Autodesk Inventor part; units mm, degrees
(part 2 of 2)
  line L983 (36.3398, 14.9098) -> (36.7208, 14.9098)
  line L984 (36.5303, 14.7193) -> (36.5303, 15.1003)
  line L985 (36.3398, 15.9918) -> (36.7208, 15.9918)
  line L986 (36.5303, 15.8013) -> (36.5303, 16.1823)
  line L987 (35.2146, 14.9098) -> (35.5956, 14.9098)
  line L988 (35.4051, 14.7193) -> (35.4051, 15.1003)
  line L989 (35.2146, 15.9918) -> (35.5956, 15.9918)
  line L990 (35.4051, 15.8013) -> (35.4051, 16.1823)
  line L991 (34.0893, 17.0713) -> (34.4703, 17.0713)
  line L992 (34.2798, 16.8808) -> (34.2798, 17.2618)
  line L993 (36.3398, 17.0713) -> (36.7208, 17.0713)
  line L994 (36.5303, 16.8808) -> (36.5303, 17.2618)
  line L995 (34.0893, 15.9918) -> (34.4703, 15.9918)
  line L996 (34.2798, 15.8013) -> (34.2798, 16.1823)
  line L997 (35.2146, 17.0713) -> (35.5956, 17.0713)
  line L998 (35.4051, 16.8808) -> (35.4051, 17.2618)
  line L999 (37.465, 17.0713) -> (37.846, 17.0713)
  line L1000 (37.6555, 16.8808) -> (37.6555, 17.2618)
  line L1001 (38.5902, 17.0713) -> (38.9712, 17.0713)
  line L1002 (38.7807, 16.8808) -> (38.7807, 17.2618)
  line L1003 (34.0893, 14.9098) -> (34.4703, 14.9098)
  line L1004 (34.2798, 14.7193) -> (34.2798, 15.1003)
  line L1005 (34.0893, 13.7617) -> (34.4703, 13.7617)
  line L1006 (34.2798, 13.5712) -> (34.2798, 13.9522)
  line L1007 (38.5902, 11.6002) -> (38.9712, 11.6002)
  line L1008 (38.7807, 11.4097) -> (38.7807, 11.7907)
  line L1009 (37.465, 11.6002) -> (37.846, 11.6002)
  line L1010 (37.6555, 11.4097) -> (37.6555, 11.7907)
  line L1011 (35.2146, 11.6002) -> (35.5956, 11.6002)
  line L1012 (35.4051, 11.4097) -> (35.4051, 11.7907)
  line L1013 (34.0893, 12.6822) -> (34.4703, 12.6822)
  line L1014 (34.2798, 12.4917) -> (34.2798, 12.8727)
  line L1015 (36.3398, 11.6002) -> (36.7208, 11.6002)
  line L1016 (36.5303, 11.4097) -> (36.5303, 11.7907)
  line L1017 (34.0893, 11.6002) -> (34.4703, 11.6002)
  line L1018 (34.2798, 11.4097) -> (34.2798, 11.7907)
  line L1019 (35.2146, 12.6822) -> (35.5956, 12.6822)
  line L1020 (35.4051, 12.4917) -> (35.4051, 12.8727)
  line L1021 (35.2146, 13.7617) -> (35.5956, 13.7617)
  line L1022 (35.4051, 13.5712) -> (35.4051, 13.9522)
  line L1023 (36.3398, 12.6822) -> (36.7208, 12.6822)
  line L1024 (36.5303, 12.4917) -> (36.5303, 12.8727)
  line L1025 (36.3398, 13.7617) -> (36.7208, 13.7617)
  line L1026 (36.5303, 13.5712) -> (36.5303, 13.9522)
  line L1027 (37.465, 12.6822) -> (37.846, 12.6822)
  line L1028 (37.6555, 12.4917) -> (37.6555, 12.8727)
  line L1029 (37.465, 13.7617) -> (37.846, 13.7617)
  line L1030 (37.6555, 13.5712) -> (37.6555, 13.9522)
  line L1031 (38.5902, 12.6822) -> (38.9712, 12.6822)
  line L1032 (38.7807, 12.4917) -> (38.7807, 12.8727)
  line L1033 (38.5902, 13.7617) -> (38.9712, 13.7617)
  line L1034 (38.7807, 13.5712) -> (38.7807, 13.9522)
  line L1035 (38.5902, 10.5207) -> (38.9712, 10.5207)
  line L1036 (38.7807, 10.3302) -> (38.7807, 10.7112)
  line L1037 (37.465, 10.5207) -> (37.846, 10.5207)
  line L1038 (37.6555, 10.3302) -> (37.6555, 10.7112)
  line L1039 (36.3398, 10.5207) -> (36.7208, 10.5207)
  line L1040 (36.5303, 10.3302) -> (36.5303, 10.7112)
  line L1041 (35.2146, 10.5207) -> (35.5956, 10.5207)
  line L1042 (35.4051, 10.3302) -> (35.4051, 10.7112)
  line L1043 (34.0893, 9.4412) -> (34.4703, 9.4412)
  line L1044 (34.2798, 9.2507) -> (34.2798, 9.6317)
  line L1045 (36.3398, 9.4412) -> (36.7208, 9.4412)
  line L1046 (36.5303, 9.2507) -> (36.5303, 9.6317)
  line L1047 (34.0893, 10.5207) -> (34.4703, 10.5207)
  line L1048 (34.2798, 10.3302) -> (34.2798, 10.7112)
  line L1049 (35.2146, 9.4412) -> (35.5956, 9.4412)
  line L1050 (35.4051, 9.2507) -> (35.4051, 9.6317)
  line L1051 (37.465, 9.4412) -> (37.846, 9.4412)
  line L1052 (37.6555, 9.2507) -> (37.6555, 9.6317)
  line L1053 (38.5902, 9.4412) -> (38.9712, 9.4412)
  line L1054 (38.7807, 9.2507) -> (38.7807, 9.6317)
  line L1055 (38.5902, 19.2303) -> (38.9712, 19.2303)
  line L1056 (38.7807, 19.0398) -> (38.7807, 19.4208)
  line L1057 (37.465, 19.2303) -> (37.846, 19.2303)
  line L1058 (37.6555, 19.0398) -> (37.6555, 19.4208)
  line L1059 (35.2146, 19.2303) -> (35.5956, 19.2303)
  line L1060 (35.4051, 19.0398) -> (35.4051, 19.4208)
  line L1061 (34.0893, 18.1508) -> (34.4703, 18.1508)
  line L1062 (34.2798, 17.9603) -> (34.2798, 18.3413)
  line L1063 (36.3398, 19.2303) -> (36.7208, 19.2303)
  line L1064 (36.5303, 19.0398) -> (36.5303, 19.4208)
  line L1065 (34.0893, 19.2303) -> (34.4703, 19.2303)
  line L1066 (34.2798, 19.0398) -> (34.2798, 19.4208)
  line L1067 (35.2146, 18.1508) -> (35.5956, 18.1508)
  line L1068 (35.4051, 17.9603) -> (35.4051, 18.3413)
  line L1069 (36.3398, 18.1508) -> (36.7208, 18.1508)
  line L1070 (36.5303, 17.9603) -> (36.5303, 18.3413)
  line L1071 (37.465, 18.1508) -> (37.846, 18.1508)
  line L1072 (37.6555, 17.9603) -> (37.6555, 18.3413)
  line L1073 (38.5902, 18.1508) -> (38.9712, 18.1508)
  line L1074 (38.7807, 17.9603) -> (38.7807, 18.3413)
  line L1075 (24.1935, 38.735) -> (24.5745, 38.735)
  line L1076 (24.384, 38.5445) -> (24.384, 38.9255)
  line L1077 (21.3995, 35.56) -> (21.7805, 35.56)
  line L1078 (21.59, 35.3695) -> (21.59, 35.7505)
  line L1079 (3.8735, 27.94) -> (4.2545, 27.94)
  line L1080 (4.064, 27.7495) -> (4.064, 28.1305)
  line L1081 (3.8735, 17.653) -> (4.2545, 17.653)
  line L1082 (4.064, 17.4625) -> (4.064, 17.8435)
  line L1083 (3.1115, 20.574) -> (3.4925, 20.574)
  line L1084 (3.302, 20.3835) -> (3.302, 20.7645)
  line L1085 (4.8895, 27.94) -> (5.2705, 27.94)
  line L1086 (5.08, 27.7495) -> (5.08, 28.1305)
  line L1087 (4.6355, 18.415) -> (5.0165, 18.415)
  line L1088 (4.826, 18.2245) -> (4.826, 18.6055)
  line L1089 (3.8735, 10.541) -> (4.2545, 10.541)
  line L1090 (4.064, 10.3505) -> (4.064, 10.7315)
  line L1091 (10.6045, 34.29) -> (10.9855, 34.29)
  line L1092 (10.795, 34.0995) -> (10.795, 34.4805)
  line L1093 (9.4615, 8.128) -> (9.8425, 8.128)
  line L1094 (9.652, 7.9375) -> (9.652, 8.3185)
  line L1095 (7.8105, 13.081) -> (8.1915, 13.081)
  line L1096 (8.001, 12.8905) -> (8.001, 13.2715)
  line L1097 (47.8155, 27.94) -> (48.1965, 27.94)
  line L1098 (48.006, 27.7495) -> (48.006, 28.1305)
  line L1099 (12.446, 26.4414) -> (12.954, 26.4414)
  line L1100 (12.7, 26.1874) -> (12.7, 26.6954)
  line L1101 (19.2405, 47.5107) -> (19.6215, 47.5107)
  line L1102 (19.431, 47.3202) -> (19.431, 47.7012)
  line L1103 (18.7325, 11.303) -> (19.1135, 11.303)
  line L1104 (18.923, 11.1125) -> (18.923, 11.4935)
  line L1105 (18.2245, 10.414) -> (18.6055, 10.414)
  line L1106 (18.415, 10.2235) -> (18.415, 10.6045)
  line L1107 (18.2245, 9.398) -> (18.6055, 9.398)
  line L1108 (18.415, 9.2075) -> (18.415, 9.5885)
  line L1109 (23.5585, 11.176) -> (23.9395, 11.176)
  line L1110 (23.749, 10.9855) -> (23.749, 11.3665)
  line L1111 (18.0975, 6.223) -> (18.4785, 6.223)
  line L1112 (18.288, 6.0325) -> (18.288, 6.4135)
  line L1113 (16.7005, 50.038) -> (17.0815, 50.038)
  line L1114 (16.891, 49.8475) -> (16.891, 50.2285)
  line L1115 (9.7155, 43.053) -> (10.0965, 43.053)
  line L1116 (9.906, 42.8625) -> (9.906, 43.2435)
  line L1117 (12.5095, 43.053) -> (12.8905, 43.053)
  line L1118 (12.7, 42.8625) -> (12.7, 43.2435)
  line L1119 (5.3975, 26.035) -> (5.7785, 26.035)
  line L1120 (5.588, 25.8445) -> (5.588, 26.2255)
  line L1121 (6.1595, 25.4) -> (6.5405, 25.4)
  line L1122 (6.35, 25.2095) -> (6.35, 25.5905)
  line L1123 (7.8105, 25.4) -> (8.1915, 25.4)
  line L1124 (8.001, 25.2095) -> (8.001, 25.5905)
  line L1125 (7.0485, 24.638) -> (7.4295, 24.638)
  line L1126 (7.239, 24.4475) -> (7.239, 24.8285)
  line L1127 (8.5725, 26.035) -> (8.9535, 26.035)
  line L1128 (8.763, 25.8445) -> (8.763, 26.2255)
  line L1129 (28.7655, 14.3358) -> (29.1465, 14.3358)
  line L1130 (28.956, 14.1453) -> (28.956, 14.5263)
  line L1131 (28.4226, -3.4544) -> (27.4091, -3.4544)
  line L1132 (27.4091, -3.4544) -> (28.4226, -2.4384)
  line L1133 (28.4226, -2.4384) -> (28.4226, -2.1844)
  line L1134 (28.4226, -2.1844) -> (28.1711, -1.9304)
  line L1135 (28.1711, -1.9304) -> (27.6631, -1.9304)
  line L1136 (27.6631, -1.9304) -> (27.4091, -2.1844)
  line L1137 (29.9466, -1.9304) -> (28.9306, -1.9304)
  line L1138 (28.9306, -1.9304) -> (28.9306, -2.6924)
  line L1139 (28.9306, -2.6924) -> (29.4386, -2.4384)
  line L1140 (29.4386, -2.4384) -> (29.6926, -2.4384)
  line L1141 (29.6926, -2.4384) -> (29.9466, -2.6924)
  line L1142 (29.9466, -2.6924) -> (29.9466, -3.2004)
  line L1143 (29.9466, -3.2004) -> (29.6926, -3.4544)
  line L1144 (29.6926, -3.4544) -> (29.1846, -3.4544)
  line L1145 (29.1846, -3.4544) -> (28.9306, -3.2004)
  line L1146 (31.4706, -1.9304) -> (30.9626, -2.1844)
  line L1147 (30.9626, -2.1844) -> (30.4546, -2.6924)
  line L1148 (30.4546, -2.6924) -> (30.4546, -3.2004)
  line L1149 (30.4546, -3.2004) -> (30.7086, -3.4544)
  line L1150 (30.7086, -3.4544) -> (31.2166, -3.4544)
  line L1151 (31.2166, -3.4544) -> (31.4706, -3.2004)
  line L1152 (31.4706, -3.2004) -> (31.4706, -2.9464)
  line L1153 (31.4706, -2.9464) -> (31.2166, -2.6924)
  line L1154 (31.2166, -2.6924) -> (30.4546, -2.6924)
  line L1155 (31.9786, -2.1844) -> (32.2326, -1.9304)
  line L1156 (32.2326, -1.9304) -> (32.7406, -1.9304)
  line L1157 (32.7406, -1.9304) -> (32.9946, -2.1844)
  line L1158 (32.9946, -2.1844) -> (32.9946, -3.2004)
  line L1159 (32.9946, -3.2004) -> (32.7406, -3.4544)
  line L1160 (32.7406, -3.4544) -> (32.2326, -3.4544)
  line L1161 (32.2326, -3.4544) -> (31.9786, -3.2004)
  line L1162 (31.9786, -3.2004) -> (31.9786, -2.1844)
  line L1163 (33.5026, -3.4544) -> (33.5026, -2.4384)
  line L1164 (33.5026, -2.4384) -> (33.7566, -2.4384)
  line L1165 (33.7566, -2.4384) -> (34.0106, -2.6924)
  line L1166 (34.0106, -2.6924) -> (34.0106, -3.4544)
  line L1167 (34.0106, -3.4544) -> (34.0106, -2.6924)
  line L1168 (34.0106, -2.6924) -> (34.2646, -2.4384)
  line L1169 (34.2646, -2.4384) -> (34.5186, -2.6924)
  line L1170 (34.5186, -2.6924) -> (34.5186, -3.4544)
  line L1171 (35.0266, -3.4544) -> (35.5346, -3.4544)
  line L1172 (35.5346, -3.4544) -> (35.2806, -3.4544)
  line L1173 (35.2806, -3.4544) -> (35.2806, -2.4384)
  line L1174 (35.2806, -2.4384) -> (35.0266, -2.4384)
  line L1175 (36.2941, -3.4544) -> (36.8021, -3.4544)
  line L1176 (36.8021, -3.4544) -> (36.5481, -3.4544)
  line L1177 (36.5481, -3.4544) -> (36.5481, -1.9304)
  line L1178 (36.5481, -1.9304) -> (36.2941, -1.9304)
  line L1179 (-1.6256, 21.5646) -> (-1.6256, 20.5511)
  line L1180 (-1.6256, 20.5511) -> (-2.6416, 21.5646)
  line L1181 (-2.6416, 21.5646) -> (-2.8956, 21.5646)
  line L1182 (-2.8956, 21.5646) -> (-3.1496, 21.3106)
  line L1183 (-3.1496, 21.3106) -> (-3.1496, 20.8051)
  line L1184 (-3.1496, 20.8051) -> (-2.8956, 20.5511)
  line L1185 (-2.8956, 22.0726) -> (-3.1496, 22.3266)
  line L1186 (-3.1496, 22.3266) -> (-3.1496, 22.8346)
  line L1187 (-3.1496, 22.8346) -> (-2.8956, 23.0886)
  line L1188 (-2.8956, 23.0886) -> (-1.8796, 23.0886)
  line L1189 (-1.8796, 23.0886) -> (-1.6256, 22.8346)
  line L1190 (-1.6256, 22.8346) -> (-1.6256, 22.3266)
  line L1191 (-1.6256, 22.3266) -> (-1.8796, 22.0726)
  line L1192 (-1.8796, 22.0726) -> (-2.8956, 22.0726)
  line L1193 (-1.6256, 24.6126) -> (-1.6256, 23.5966)
  line L1194 (-1.6256, 23.5966) -> (-2.6416, 24.6126)
  line L1195 (-2.6416, 24.6126) -> (-2.8956, 24.6126)
  line L1196 (-2.8956, 24.6126) -> (-3.1496, 24.3586)
  line L1197 (-3.1496, 24.3586) -> (-3.1496, 23.8506)
  line L1198 (-3.1496, 23.8506) -> (-2.8956, 23.5966)
  line L1199 (-2.8956, 25.1206) -> (-3.1496, 25.3746)
  line L1200 (-3.1496, 25.3746) -> (-3.1496, 25.8826)
  line L1201 (-3.1496, 25.8826) -> (-2.8956, 26.1366)
  line L1202 (-2.8956, 26.1366) -> (-1.8796, 26.1366)
  line L1203 (-1.8796, 26.1366) -> (-1.6256, 25.8826)
  line L1204 (-1.6256, 25.8826) -> (-1.6256, 25.3746)
  line L1205 (-1.6256, 25.3746) -> (-1.8796, 25.1206)
  line L1206 (-1.8796, 25.1206) -> (-2.8956, 25.1206)
  line L1207 (-1.6256, 26.6446) -> (-2.6416, 26.6446)
  line L1208 (-2.6416, 26.6446) -> (-2.6416, 26.8986)
  line L1209 (-2.6416, 26.8986) -> (-2.3876, 27.1526)
  line L1210 (-2.3876, 27.1526) -> (-1.6256, 27.1526)
  line L1211 (-1.6256, 27.1526) -> (-2.3876, 27.1526)
  line L1212 (-2.3876, 27.1526) -> (-2.6416, 27.4066)
  line L1213 (-2.6416, 27.4066) -> (-2.3876, 27.6606)
  line L1214 (-2.3876, 27.6606) -> (-1.6256, 27.6606)
  line L1215 (-1.6256, 28.1686) -> (-1.6256, 28.6766)
  line L1216 (-1.6256, 28.6766) -> (-1.6256, 28.4226)
  line L1217 (-1.6256, 28.4226) -> (-2.6416, 28.4226)
  line L1218 (-2.6416, 28.4226) -> (-2.6416, 28.1686)
  line L1219 (-1.6256, 29.4361) -> (-1.6256, 29.9441)
  line L1220 (-1.6256, 29.9441) -> (-1.6256, 29.6901)
  line L1221 (-1.6256, 29.6901) -> (-3.1496, 29.6901)
  line L1222 (-3.1496, 29.6901) -> (-3.1496, 29.4361)
  line L1223 (0, 51.308) -> (65.024, 51.308)
  line L1224 (65.024, 0) -> (3.81, 0)
  line L1225 (0, 33.8582) -> (0, 51.308)
  circle A0 centre (3.81, 47.244) radius 1.6
  circle A1 centre (11.43, 4.064) radius 1.6
  line L1226 (0, 51.308) -> (-1, 51.308)
  line L1227 (65.024, 51.308) -> (66.024, 51.308)
  line L1228 (-1, 51.308) -> (66.024, 51.308)
  line L1229 (66.024, 0) -> (3.81, 0)
  line L1230 (64.008, 40.9473) -> (58.42, 40.9473)
  line L1231 (58.42, 40.9473) -> (58.42, 9.5961)
  line L1232 (58.42, 9.5961) -> (64.008, 9.5961)
  line L1233 (64.008, 9.5961) -> (64.008, 40.9473)
  line L1234 (-1, 34.3967) -> (-1, 33.8582)
  line L1235 (3.81, 0) -> (6.3805, 0)
  line L1236 (6.3805, 13.5712) -> (6.3805, 34.3967)
  line L1237 (32.512, 51.308) -> (6.3805, 51.308)
  line L1238 (6.3805, 13.5712) -> (32.512, 13.5712)
  line L1239 (32.512, 40.9228) -> (6.3805, 40.9228)
  line L1240 (6.3805, 35.6667) -> (32.512, 35.6667)
  line L1241 (32.512, 13.5712) -> (32.512, 35.6667)
  line L1242 (32.512, 40.9228) -> (32.512, 48.844)
  line L1243 (6.3805, 48.844) -> (6.3805, 40.9228)
  line L1244 (6.3805, 35.6667) -> (6.3805, 13.5712)
  line L1245 (32.512, 48.844) -> (6.3805, 48.844)
  line L1246 (51.308, 48.844) -> (34.2798, 48.844)
  line L1247 (34.2798, 48.844) -> (34.2798, 29.9441)
  line L1248 (34.2798, 29.9441) -> (51.308, 29.9441)
  line L1249 (51.308, 29.9441) -> (51.308, 48.844)
  line L1250 (51.308, 22.8346) -> (34.2798, 22.8346)
  line L1251 (34.2798, 22.8346) -> (34.2798, 4.6863)
  line L1252 (34.2798, 4.6863) -> (51.308, 4.6863)
  line L1253 (51.308, 4.6863) -> (51.308, 22.8346)
  line L1254 (-1, 7.6276) -> (-2.2, 7.6276)
  line L1255 (3.81, 33.8582) -> (-1, 33.8582)
  line L1256 (3.81, 0) -> (3.81, 33.8582)
  line L1257 (-1, 33.8582) -> (-1, 51.308)
  line L1258 (0, 55.1688) -> (0, -3.4544) construction
  line L1259 (66.024, 9.1526) -> (67.024, 9.1526)
  line L1260 (67.024, 9.1526) -> (67.024, 15.1526)
  line L1261 (67.024, 15.1526) -> (66.024, 15.1526)
  line L1262 (66.024, 9.1526) -> (67.024, 9.1526)
  line L1263 (67.024, 9.1526) -> (67.024, 15.1526)
  line L1264 (67.024, 15.1526) -> (66.024, 15.1526)
  line L1265 (66.024, 51.308) -> (66.024, 15.1526)
  line L1266 (66.024, 9.1526) -> (66.024, 0)
  point P0 (0, 0)
  point P1 (0, 0)
  point P2 (66.024, 7.6276)
  dimension "d0" = 65.024
  dimension "d1" = 3.2
  dimension "d2" = 3.2
  dimension "d5" = 1
  dimension "d6" = 1
  constraints: 2534 end point, 17 parallel, 10 horizontal, 7 perpendicular, 5 point on line, 3 midpoint, 2 centre point, 1 vertical
  measures "d0" distance between parallel lines of L18 L16
  measures "d1" diameter of A0
  measures "d2" diameter of A1
  measures "d5" distance of L1225.end L1226.end
  measures "d6" distance of L1223.end L1227.end
extrude "押し出し3" add sketch "スケッチ1" along normal blind 3 contours L8 L1226 L16 L1255 L1234 L1257 | L17 L18 L19 L1256 L1255 L16 | L1227 L1265 L1261 L1260 L1259 L1266 L1229 L18
sketch "スケッチ2" plane through (0, 0, 0) normal (0, 0, -1) x (-1, 0, 0)
  line L0 (-66.024, 0) -> (-66.024, 51.308) projected
  line L1 (-66.024, 9.1526) -> (-67.024, 9.1526)
  line L2 (-67.024, 9.1526) -> (-67.024, 15.1526)
  line L3 (-67.024, 15.1526) -> (-66.024, 15.1526)
  line L4 (-66.024, 15.1526) -> (-66.024, 9.1526)
  line L5 (-66.024, 15.1526) -> (-65.024, 15.1526)
  line L6 (-65.024, 15.1526) -> (-65.024, 9.1526)
  line L7 (-65.024, 9.1526) -> (-66.024, 9.1526)
  line L8 (-66.024, 9.1526) -> (-66.024, 15.1526)
  point P0 (0, 0)
  dimension "d14" = 1
  dimension "d15" = 6
  dimension "d16" = 1
  constraints: 16 end point, 4 parallel, 2 horizontal, 2 perpendicular, 1 point on line
  measures "d14" distance of L2.end L3.end
  measures "d15" distance of L1.end L2.end
  measures "d16" distance of L6.end L7.end
extrude "押し出し4" add sketch "スケッチ2" along normal blind 12
chamfer "面取り1" distance 1 angle 45 3 edges at (65.024, 12.1526, 0) (65.524, 15.1526, 0) (65.524, 9.1526, 0)
chamfer "面取り2" distance 1 angle 45 4 edges at (66.024, 9.1526, -0.5) (66.024, 9.1526, 1.5) (66.024, 15.1526, -0.5) (66.024, 15.1526, 1.5)
chamfer "面取り3" distance 1 angle 45 10 edges at (64.008, 40.9473, 1.5) (51.308, 48.844, 1.5) (32.512, 48.844, 1.5) (32.512, 35.6667, 1.5) (51.308, 29.9441, 1.5) (32.512, 40.9228, 1.5) (32.512, 13.5712, 1.5) (64.008, 9.5961, 1.5) (58.42, 9.5961, 1.5) (6.3805, 13.5712, 1.5)
chamfer "面取り4" distance 1 angle 45 7 edges at (34.2798, 48.844, 1.5) (6.3805, 48.844, 1.5) (6.3805, 35.6667, 1.5) (34.2798, 22.8346, 1.5) (34.2798, 29.9441, 1.5) (34.2798, 4.6863, 1.5) (6.3805, 40.9228, 1.5)
chamfer "面取り5" distance 1 angle 45 6 edges at (51.308, 4.6863, 1.5) (51.308, 22.8346, 1.5) (58.42, 40.9473, 1.5) (3.81, 33.8582, 1.5) (66.024, 15.1526, -12) (66.024, 9.1526, -12)
sketch "スケッチ3" plane through (65.024, 9.1526, -1) normal (-1, 0, 0) x (0, 0, 1)
  circle A0 centre (-7.5, 3) radius 2.1
  line L0 (1, 23.7056) -> (1, -9.1526) projected
  line L1 (0, 6) -> (-10, 6) projected
  dimension "d40" = 4.2
  dimension "d41" = 8.5
  dimension "d42" = 3
  constraints: 1 centre point
  measures "d40" diameter of A0
  measures "d41" distance from line of L0 A0.centre
  measures "d42" distance from line of L1 A0.centre
extrude "押し出し5" cut sketch "スケッチ3" against normal blind 2
